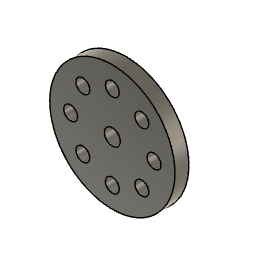
gripper_ (Autodesk Fusion 360 archive; units mm, degrees)
design "new gripper_servo horn"
Autodesk Fusion 360 part; units mm, degrees
sketch "스케치1" plane through (0, 0, 0) normal (0, 1, 0) x (1, 0, 0)
  circle A0 centre (0, 0) radius 9
  circle A1 centre (0, 0) radius 2.5
  circle A2 centre (0, 0) radius 6 construction
  circle A3 centre (6, 0) radius 1
  circle A4 centre (4.2426, 4.2426) radius 1
  circle A5 centre (0, 6) radius 1
  circle A6 centre (-4.2426, 4.2426) radius 1
  circle A7 centre (-6, 0) radius 1
  circle A8 centre (-4.2426, -4.2426) radius 1
  circle A9 centre (0, -6) radius 1
  circle A10 centre (4.2426, -4.2426) radius 1
  circle A11 centre (0, 0) radius 1.15
  circle A12 centre (0, 0) radius 2.2
  circle A13 centre (0, 0) radius 3.5
  dimension "d1" = 18
  dimension "d2" = 5
  dimension "d3" = 12
  dimension "d4" = 2
  dimension "d6" = 360
  dimension "d7" = 2.3
  dimension "d10" = 4.4
  dimension "d11" = 7
  constraint coincident A0.centre A1.centre
  constraint concentric A0 A1
  constraint coincident A2 A3.centre
  constraint concentric A1 A11
  constraint concentric A11 A12
  constraint concentric A11 A13
  measures "d1" diameter of A0
  measures "d2" diameter of A1
  measures "d3" diameter of A2
  measures "d4" diameter of A3
  measures "d7" diameter of A11
  measures "d10" diameter of A12
  measures "d11" diameter of A13
extrude "돌출1" add sketch "스케치1" against normal blind 2 contours A0 | A1 | A12 | A13
extrude "돌출2" add sketch "스케치1" along normal blind 2.5 contours A1 | A13
